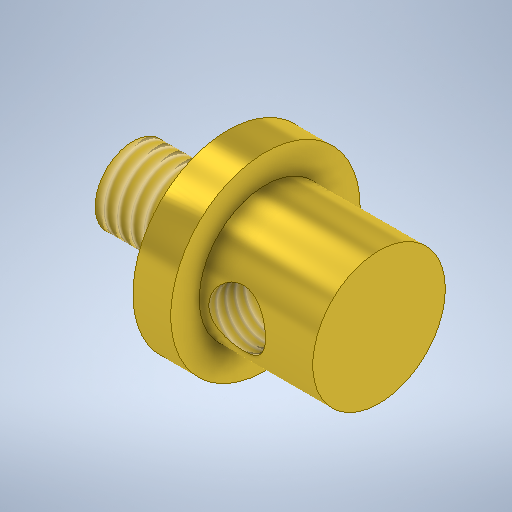
# Autodesk Inventor part: 134
Saved by Autodesk Inventor 2025.1 (Build 291241000, 241)
## iProperties
Created: 2024-08-05
Part Number: 134
Material: Lead
Document SubType Name: Modeling
Designer: ffogue
Density: 11.34 g/cm^3
Appearance: Metal 2400F Hot
Author: ffogue
Autodesk Inventor part; units mm, degrees
ref_plane "YZ Plane" through (0, 0, 0) normal (1, 0, 0) x (0, 1, 0)
ref_plane "XY Plane" through (0, 0, 0) normal (0, 0, 1) x (1, 0, 0)
sketch "Sketch1" plane through (0, 0, 0) normal (0, 0, 1) x (1, 0, 0)
  line L0 (0, 0) -> (0, 2)
  line L1 (0, 2) -> (5, 2)
  line L2 (5, 2) -> (5, 5)
  line L3 (5, 5) -> (7, 5)
  line L4 (7, 5) -> (7, 3.5)
  line L5 (7, 3.5) -> (13, 3.5)
  line L6 (13, 3.5) -> (13, 0)
  line L7 (13, 0) -> (0, 0)
  point P0 (10, 3.5)
  dimension "d0" = 4
  dimension "d1" = 5
  dimension "d2" = 2
  dimension "d3" = 10
  dimension "d4" = 7
  dimension "d5" = 6
  constraints: 16 end point, 7 perpendicular, 1 midpoint, 1 vertical
  measures "d0" diameter of L1 L7
  measures "d1" distance of L0.end L1.end
  measures "d2" distance of L2.end L3.end
  measures "d3" diameter of L3 L7
  measures "d4" diameter of point (10, 3.5) L7
  measures "d5" distance of L4.end L5.end
revolve "Revolution1" add sketch "Sketch1" angle 360 about axis through (13, 0, 0) along (-1, 0, 0)
thread "Thread1" size "M4x0.7" class "6g" standard "ISO Metric profile" length 10
ref_plane "Work Plane3" through (0, -3.5, 0) normal (0, 1, 0) x (-1, 0, 0)
sketch "Sketch5" plane through (0, -3.5, 0) normal (0, 1, 0) x (-1, 0, 0)
  line L0 (-13, -3.5) -> (-13, 3.5) projected
  point P0 (0, 0)
  point P1 (-9, 0)
  dimension "d13" = 4
  constraints: 1 horizontal alignment
  measures "d13" distance from line of L0 point (-9, 0)
hole "Hole1" at (9, -3.5, 0) direction (0, 1, 0) diameter 3 depth 2.5
thread "Thread2" size "M3x0.5" class "6H" standard "ISO Metric profile" length 10
body "Solid1"
